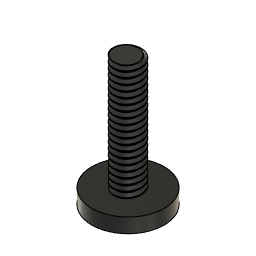
螺丝 v1 v1 (Autodesk Fusion 360 design; units mm, degrees)
Autodesk Fusion 360 part; units mm, degrees
sketch "草图1" plane through (0, 0, 0) normal (0, 0, 1) x (1, 0, 0)
  circle A0 centre (0, 0) radius 2.5
  dimension "d1" = 5
  constraint coincident A0.centre origin
  measures "d1" diameter of A0
extrude "拉伸1" add sketch "草图1" along normal blind 1
sketch "草图2" plane through (0, 0, 0) normal (0, 0, -1) x (1, 0, 0)
  circle A0 centre (0, 0) radius 2.5
  line L0 (2, 0) -> (1, 1.7321)
  line L1 (1, 1.7321) -> (-1, 1.7321)
  line L2 (-1, 1.7321) -> (-2, 0)
  line L3 (-2, 0) -> (-1, -1.7321)
  line L4 (-1, -1.7321) -> (1, -1.7321)
  line L5 (1, -1.7321) -> (2, 0)
  dimension "d4" = 2
  constraint coincident A0.centre origin
  measures "d4" distance of L0.start A0.centre
extrude "拉伸2" cut sketch "草图2" against normal blind 0.5 contours L0 L1 L2 L3 L4 L5
sketch "草图3" plane through (0, 0, 1) normal (0, 0, 1) x (-1, 0, 0)
  circle A0 centre (0, 0) radius 2.5
  circle A1 centre (0, 0) radius 1
  dimension "d7" = 2
  constraint coincident A0.centre A1.centre
  measures "d7" diameter of A1
extrude "拉伸3" add sketch "草图3" along normal blind 8 contours A1
thread "螺纹1" "ISO Metric profile 2.0 M2x0.4 6g" major diameter 1.9335 minor diameter 1.478 pitch 0.4 angle 60 modelled right hand crest width 0.058 on face at (-0.9988, 0.0498, 6.3333) crest through (-0.9668, 0, 0.9)
